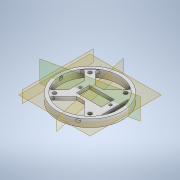
# Autodesk Inventor part: Servo_holder
Saved by Autodesk Inventor 2020 (Build 240168000, 168)
## iProperties
Created: 2020-09-03
Part Number: Servo_holder
Material: Generisch
Document SubType Name: Modeling
Designer: sp
Density: 1 g/cm^3
Appearance: Vorgabe
Author: sp
## iProperties of the stored document _3D-Druck.ipt
Created: 2020-09-03
Part Number: _3D-Druck
Material: Generisch
Document SubType Name: Modeling
Designer: sp
Density: 1 g/cm^3
Appearance: Vorgabe
Author: sp
Autodesk Inventor part; units mm, degrees
ref_plane "XY Plane" through (0, 0, 0) normal (0, 0, 1) x (1, 0, 0)
sketch "Skizze1" plane through (0, 0, 0) normal (0, 1, 0) x (-1, 0, 0)
  circle A0 centre (0, 0) radius 30
  circle A1 centre (0, 0) radius 27
  dimension "d0" = 60
  dimension "d1" = 54
  constraints: 2 centre point, 2 coincident
  measures "d0" diameter of A0
  measures "d1" diameter of A1
extrude "Extrusion1" add sketch "Skizze1" along normal mid plane 10
ref_plane "Arbeitsebene1" through (0, 0, 0) normal (0, 1, 0) x (-1, 0, 0)
sketch "Skizze2" plane through (0, 0, 0) normal (0, 1, 0) x (-1, 0, 0)
  line L0 (0, 42.2301) -> (0, -36.7007) construction
  line L1 (32.6355, 0) -> (-32.6355, 0) construction
  line L2 (16.5, 34.419) -> (16.5, -40.3324) construction
  line L3 (-16.5, 35.4304) -> (-16.5, -34.8157) construction
  line L4 (23.5881, 16.5) -> (-32.0387, 16.5) construction
  line L5 (23.5881, -16.5) -> (-39.8541, -16.5) construction
  circle A0 centre (16.5, -16.5) radius 1.75
  circle A1 centre (16.5, 16.5) radius 1.75
  circle A2 centre (-16.5, 16.5) radius 1.75
  circle A3 centre (-16.5, -16.5) radius 1.75
  circle A4 centre (-16.5, 16.5) radius 3.6749
  circle A5 centre (-16.5, -16.5) radius 3.7161
  circle A6 centre (16.5, -16.5) radius 3.7
  circle A7 centre (16.5, 16.5) radius 3.6747
  point P0 (0, 0)
  dimension "d8" = 33
  dimension "d9" = 33
  dimension "d10" = 3.5
  dimension "d11" = 3.5
  dimension "d12" = 3.5
  dimension "d13" = 3.5
  constraints: 12 end point, 9 point on line, 8 centre point, 4 coincident, 3 horizontal, 3 vertical, 1 midpoint, 2 other
  measures "d8" distance between parallel lines of L3 L2
  measures "d9" distance between parallel lines of L4 L5
  measures "d10" diameter of A0
  measures "d11" diameter of A1
  measures "d12" diameter of A2
  measures "d13" diameter of A3
extrude "Extrusion2" add sketch "Skizze2" along normal mid plane 3
fillet "Rundung1" radius 2 16 edges at (-18.7043, 0.75, -19.4718) (-19.4718, 0.75, -18.7043) (-18.7043, -0.75, -19.4718) (-19.4718, -0.75, -18.7043) (-19.289, 0.75, 18.8927) (-18.8927, 0.75, 19.289) (-19.289, -0.75, 18.8927) (-18.8927, -0.75, 19.289) (18.8904, 0.75, 19.2913) (19.2913, 0.75, 18.8904) (18.8904, -0.75, 19.2913) (19.2913, -0.75, 18.8904) (19.551, 0.75, -18.6215) (18.6215, 0.75, -19.551) (19.551, -0.75, -18.6215) (18.6215, -0.75, -19.551)
sketch "Skizze3" plane through (0, 0, 0) normal (0, 1, 0) x (-1, 0, 0)
  line L0 (38.199, 0) -> (-35.7579, 0) construction
  line L1 (0, -41.7977) -> (0, 48.2137) construction
  line L2 (6.5, -6) -> (-16.5, -6)
  line L3 (-16.5, -6) -> (-16.5, 6)
  line L4 (-16.5, 6) -> (6.5, 6)
  line L5 (6.5, 6) -> (6.5, -6)
  arc A0 (14.419, 19.5287) -> (19.5287, 14.419) centre (16.5, 16.5) ccw projected
  arc A1 (-14.386, -19.5562) -> (-19.5562, -14.386) centre (-16.5, -16.5) ccw projected
  line L6 (19.5287, 14.419) -> (-14.386, -19.5562)
  line L7 (13.9016, 19.0984) -> (-19.1253, -13.87)
  arc A2 (19.5455, -14.3988) -> (14.3988, -19.5455) centre (16.5, -16.5) ccw projected
  arc A3 (-19.5289, 14.4189) -> (-14.4189, 19.5289) centre (-16.5, 16.5) ccw projected
  line L8 (19.5455, -14.3988) -> (-14.4189, 19.5289)
  line L9 (14.132, -19.3431) -> (-19.0991, 13.902)
  arc A4 (-19.5289, 14.4189) -> (-22.8714, 14.3491) centre (-21.1772, 13.2862) ccw projected
  line L10 (12.6716, -7.5323) -> (12.6716, 7.5497)
  circle A5 centre (9, 0) radius 1.25
  circle A6 centre (-19, 0) radius 1.25
  line L11 (-22.8714, 14.3491) -> (-22.8714, -14.3491)
  circle A7 centre (0, 0) radius 27 projected
  circle A8 centre (16.5, 16.5) radius 3.6747
  circle A9 centre (-16.5, -16.5) radius 3.7161
  circle A10 centre (-16.5, 16.5) radius 1.75 projected
  circle A11 centre (-16.5, 16.5) radius 3.6749
  circle A12 centre (16.5, -16.5) radius 3.6
  arc A13 (-22.8971, -14.3081) -> (-19.5562, -14.386) centre (-21.201, -13.2483) ccw projected
  circle A14 centre (-21.201, -13.2483) radius 2
  circle A15 centre (-21.1772, 13.2862) radius 2
  line L12 (3.6165, -8.8232) -> (-3.6721, -8.8232)
  line L13 (3.6165, 8.8316) -> (-3.71, 8.8316)
  point P0 (18.5864, 13.475)
  point P1 (-13.4734, 18.5844)
  point P2 (-22.8714, 14.3491)
  point P3 (-22.8714, 12.2233)
  point P4 (-22.8714, -12.1484)
  point P5 (-13.4401, -18.6085)
  point P6 (13.5202, -18.731)
  point P7 (13.8837, -13.8837)
  point P8 (18.5979, -13.4522)
  point P9 (18.517, -13.3714)
  point P10 (13.656, -18.8668)
  dimension "d17" = 12
  dimension "d18" = 23
  dimension "d19" = 6.5
  dimension "d20" = 2.5
  dimension "d21" = 2.5
  dimension "d22" = 2.5
  dimension "d23" = 2.5
  dimension "d44" = 7.2
  constraints: 28 end point, 10 point on line, 8 centre point, 6 coincident, 5 point on circle, 3 concentric, 3 parallel, 3 vertical, 2 horizontal, 2 perpendicular, 2 tangent, 1 other
  measures "d17" distance of L2.end L3.end
  measures "d18" distance of L2.start L2.end
  measures "d19" distance between parallel lines of L1 L5
  measures "d20" diameter of A6
  measures "d21" diameter of A5
  measures "d22" distance from line of A5.centre L5
  measures "d23" distance from line of L3 A6.centre
  measures "d44" diameter of A12
extrude "Extrusion3" add sketch "Skizze3" along normal mid plane 3 contours L5 L8 A2 L9 L2 | L9 L12 L6 L2 | L5 L6 L10 L8 | L6 A1 L7 L2 | L5 L4 L7 A0 L6 | L7 A1 A14 L11 A15 A3 L9 L4 L3 L2 | L9 A3 L8 L4 | L4 L8 L13 L7 | A13 L11 A14 | A7 A14 L11 | A15 L11 A4 | L11 A15
ref_plane "Arbeitsebene2" through (0, 0, 0) normal (0.9781476, 0, -0.2079117) x (0, 1, 0)
ref_plane "Arbeitsebene3" through (0, 0, 0) normal (-0.2079117, 0, -0.9781476) x (0, 1, 0)
ref_plane "Arbeitsebene4" through (-30, 0, 0) normal (1, 0, 0) x (0, 1, 0)
sketch "Skizze6" plane through (-30, 0, 0) normal (1, 0, 0) x (0, 1, 0)
  circle A0 centre (0, 0) radius 1.75
  dimension "d46" = 3.5
  constraints: 1 centre point, 1 coincident
  measures "d46" diameter of A0
extrude "Extrusion5" cut sketch "Skizze6" along normal blind 4
pattern_circular "Runde Anordnung1" count 3 over 360 about axis through (0, -10, 0) along (0, 1, 0) of "Extrusion5"
sketch "Skizze7" plane through (-30, 0, 0) normal (1, 0, 0) x (0, 1, 0)
  line L0 (5, -30) -> (5, 30) projected
  line L1 (-5, 30) -> (5, 30) projected
  line L2 (5, -30) -> (1.9826, -30)
  line L3 (1.9826, -30) -> (1.9826, 30)
  line L4 (1.9826, 30) -> (5, 30)
  line L5 (5, 30) -> (5, -30)
  point P0 (0, 0)
  constraints: 8 end point, 2 parallel, 1 horizontal, 1 perpendicular, 1 point on line
extrude "Extrusion6" cut sketch "Skizze7" along normal blind 62
